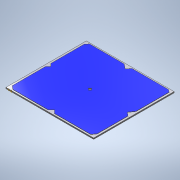
# Autodesk Inventor part: panelSolar
Saved by Autodesk Inventor 2020 (Build 240168000, 168)
## iProperties
Created: 2021-12-16
Part Number: panelSolar
Material: Genérico
Document SubType Name: Modeling
Designer: DANIEL
Density: 1 g/cm^3
Appearance: Textura fina - Negro
Author: DANIEL
Autodesk Inventor part; units mm, degrees
ref_plane "YZ Plane" through (0, 0, 0) normal (1, 0, 0) x (0, 1, 0)
ref_plane "XZ Plane" through (0, 0, 0) normal (0, 1, 0) x (-1, 0, 0)
ref_plane "XY Plane" through (0, 0, 0) normal (0, 0, 1) x (1, 0, 0)
sketch "Boceto1" plane through (0, 0, 0) normal (0, 1, 0) x (-1, 0, 0)
  line L0 (180, 165) -> (-180, 165)
  line L1 (-180, 165) -> (-180, -165)
  line L2 (-180, -165) -> (180, -165)
  line L3 (180, -165) -> (180, 165)
  point P0 (0, 0)
  dimension "ancho" = 330
  dimension "largo" = 360
  dimension "d2" = 165
  dimension "d3" = 180
  constraints: 8 end point, 2 parallel, 1 horizontal, 1 perpendicular
  measures "ancho" distance between parallel lines of L2 L0
  measures "largo" distance between parallel lines of L1 L3
  measures "d2" distance from line of L0 point (0, 0)
  measures "d3" distance from line of L3 point (0, 0)
extrude "Extrusión1" add sketch "Boceto1" along normal blind 5
sketch "Boceto3" plane through (0, 5, 0) normal (0, 1, 0) x (1, 0, 0)
  line L0 (-161.9145, -155.4161) -> (-171.724, -147.3901)
  line L1 (-171.724, -147.3901) -> (-171.724, -10.9202)
  line L2 (-180, -165) -> (180, -165) projected
  line L3 (-171.724, 10.8511) -> (-171.724, 147.7886)
  line L4 (-171.724, 147.7886) -> (-161.9145, 159.7781)
  line L5 (-161.9145, 159.7781) -> (-19.2299, 159.7781)
  line L6 (-19.2299, 159.7781) -> (0, 144.0446)
  line L7 (0, 144.0446) -> (12.8729, 159.7781)
  line L8 (12.8729, 159.7781) -> (162.2701, 159.7781)
  line L9 (162.2701, 159.7781) -> (173.0193, 151.9113)
  line L10 (173.0193, 151.9113) -> (173.0193, 15.5106)
  line L11 (180, -165) -> (180, 165) projected
  line L12 (173.0193, 15.5106) -> (158.133, -4.8303)
  line L13 (158.133, -4.8303) -> (173.0193, -17.01)
  line L14 (173.0193, -17.01) -> (173.0193, -143.5188)
  line L15 (173.0193, -143.5188) -> (161.6681, -159.0293)
  line L16 (161.6681, -159.0293) -> (12.8729, -159.0293)
  line L17 (-28.9067, -159.0293) -> (-157.4983, -159.0293)
  line L18 (-157.4983, -159.0293) -> (-161.9145, -155.4161)
  line L19 (0, -6.4152) -> (-5.5701, -0.8451)
  line L20 (0, -6.4152) -> (7.8773, -6.4152) construction
  line L21 (-5.5701, -0.8451) -> (-6.4152, 0)
  line L22 (-6.4152, 0) -> (0, 6.4152)
  line L23 (0, 6.4152) -> (6.4152, 0)
  line L24 (6.4152, 0) -> (0, -6.4152)
  line L25 (12.8729, -159.0293) -> (3.2076, -149.364)
  line L26 (12.8729, -159.0293) -> (26.5417, -159.0293) construction
  line L27 (3.2076, -149.364) -> (0, -146.1564)
  line L28 (0, -146.1564) -> (-12.8729, -159.0293)
  line L29 (-12.8729, -159.0293) -> (-28.9067, -159.0293)
  line L30 (-171.724, 10.8511) -> (-161.9145, 1.0415)
  line L31 (-171.724, 10.8511) -> (-157.8512, 10.8511) construction
  line L32 (-161.9145, 1.0415) -> (-160.8729, 0)
  line L33 (-160.8729, 0) -> (-171.724, -10.9202)
  point P0 (0, 0)
  dimension "d7" = 135
  dimension "d8" = 135
  dimension "d9" = 45
  constraints: 64 end point, 10 point on line, 8 perpendicular, 5 horizontal, 4 parallel, 3 equal length
  measures "d7" angle of L20 L19
  measures "d8" angle of L26 L25
  measures "d9" angle of L30 L31
extrude "Extrusión2" add sketch "Boceto3" along normal blind 1
equation "\"d2\" = 0.5 * ancho"
equation "\"d3\" = 0.5 * largo"
